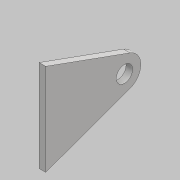
# Autodesk Inventor part: exercise3-17
Saved by Autodesk Inventor 2018 (Build 220112000, 112)
## iProperties
Created: 2020-09-23
Part Number: exercise3-17
Material: 一般
Document SubType Name: Modeling
Designer: 王鼎鈞
Density: 1 g/cm^3
Appearance: 預設
Author: 王鼎鈞
Autodesk Inventor part; units mm, degrees
ref_plane "YZ Plane" through (0, 0, 0) normal (1, 0, 0) x (0, 1, 0)
ref_plane "XZ Plane" through (0, 0, 0) normal (0, 1, 0) x (-1, 0, 0)
ref_plane "XY Plane" through (0, 0, 0) normal (0, 0, 1) x (1, 0, 0)
sketch "草圖1" plane through (0, 0, 0) normal (1, 0, 0) x (0, 1, 0)
  circle A0 centre (0, 0) radius 25
  arc A1 (17.0102, -47.0176) -> (0, 50) centre (0, 0) ccw
  line L0 (-299.5508, 0) -> (117.3046, 0) projected
  line L1 (0, -196) -> (0, 196) projected
  line L2 (-240, 140) -> (-240, -140)
  line L3 (-240, 140) -> (17.0102, 47.0176)
  line L4 (-240, -140) -> (17.0102, -47.0176)
  dimension "d0" = 50
  dimension "d1" = 100
  dimension "d2" = 280
  dimension "d3" = 240
  dimension "d4" = 140
  constraints: 6 end point, 3 point on circle, 2 centre point, 2 coincident, 2 tangent, 1 point on line, 1 vertical
  measures "d0" diameter of A0
  measures "d1" diameter of A1
  measures "d2" distance of L2.start L2.end
  measures "d3" distance between parallel lines of L1 L2
  measures "d4" distance from line of L0 L2.start
extrude "擠出1" add sketch "草圖1" along normal blind 20 contours L0 A1 L4 L1 A0 | A0 L1 A1 L0 | A0 L0 L2 L3 L1 | L1 L4 L2 L0 A0 | L1 L3 A1
